Autodesk Inventor part; units mm, degrees
(part 3 of 3)
sketch "Sketch7" plane through (0, 0, 2.286) normal (0, 0, 1) x (1, 0, 0)
  arc A0 (-117.475, -252.4125) -> (-119.38, -258.1275) centre (-117.475, -255.5875) ccw projected
  line L0 (-79.375, -252.4125) -> (-117.475, -252.4125) projected
  arc A1 (-76.2, -255.5875) -> (-79.375, -252.4125) centre (-79.375, -255.5875) ccw projected
  line L1 (-76.2, -284.1625) -> (-76.2, -255.5875) projected
  arc A2 (-81.28, -286.7025) -> (-76.2, -284.1625) centre (-79.375, -284.1625) ccw projected
  line L2 (-119.38, -258.1275) -> (-81.28, -286.7025) projected
  arc A3 (-127, 290.5125) -> (-121.92, 287.9725) centre (-123.825, 290.5125) ccw projected
  line L3 (-127, 319.0875) -> (-127, 290.5125) projected
  arc A4 (-123.825, 322.2625) -> (-127, 319.0875) centre (-123.825, 319.0875) ccw projected
  line L4 (-85.725, 322.2625) -> (-123.825, 322.2625) projected
  arc A5 (-83.82, 316.5475) -> (-85.725, 322.2625) centre (-85.725, 319.0875) ccw projected
  line L5 (-121.92, 287.9725) -> (-83.82, 316.5475) projected
  arc A6 (-180.975, 322.2625) -> (-182.88, 316.5475) centre (-180.975, 319.0875) ccw projected
  line L6 (-142.875, 322.2625) -> (-180.975, 322.2625) projected
  arc A7 (-139.7, 319.0875) -> (-142.875, 322.2625) centre (-142.875, 319.0875) ccw projected
  line L7 (-139.7, 290.5125) -> (-139.7, 319.0875) projected
  arc A8 (-144.78, 287.9725) -> (-139.7, 290.5125) centre (-142.875, 290.5125) ccw projected
  line L8 (-182.88, 316.5475) -> (-144.78, 287.9725) projected
  arc A9 (-142.875, 201.6125) -> (-139.7, 204.7875) centre (-142.875, 204.7875) ccw projected
  line L9 (-180.975, 201.6125) -> (-142.875, 201.6125) projected
  arc A10 (-182.88, 207.3275) -> (-180.975, 201.6125) centre (-180.975, 204.7875) ccw projected
  line L10 (-144.78, 235.9025) -> (-182.88, 207.3275) projected
  arc A11 (-139.7, 233.3625) -> (-144.78, 235.9025) centre (-142.875, 233.3625) ccw projected
  line L11 (-139.7, 204.7875) -> (-139.7, 233.3625) projected
  arc A12 (-85.725, 201.6125) -> (-83.82, 207.3275) centre (-85.725, 204.7875) ccw projected
  line L12 (-123.825, 201.6125) -> (-85.725, 201.6125) projected
  arc A13 (-127, 204.7875) -> (-123.825, 201.6125) centre (-123.825, 204.7875) ccw projected
  line L13 (-127, 233.3625) -> (-127, 204.7875) projected
  arc A14 (-121.92, 235.9025) -> (-127, 233.3625) centre (-123.825, 233.3625) ccw projected
  line L14 (-83.82, 207.3275) -> (-121.92, 235.9025) projected
  arc A15 (200.025, 322.2625) -> (198.12, 316.5475) centre (200.025, 319.0875) ccw projected
  line L15 (238.125, 322.2625) -> (200.025, 322.2625) projected
  arc A16 (241.3, 319.0875) -> (238.125, 322.2625) centre (238.125, 319.0875) ccw projected
  line L16 (241.3, 290.5125) -> (241.3, 319.0875) projected
  arc A17 (236.22, 287.9725) -> (241.3, 290.5125) centre (238.125, 290.5125) ccw projected
  line L17 (198.12, 316.5475) -> (236.22, 287.9725) projected
  arc A18 (-190.5, 271.4625) -> (-187.325, 268.2875) centre (-187.325, 271.4625) ccw projected
  line L18 (-190.5, 300.0375) -> (-190.5, 271.4625) projected
  arc A19 (-185.42, 302.5775) -> (-190.5, 300.0375) centre (-187.325, 300.0375) ccw projected
  line L19 (-147.32, 274.0025) -> (-185.42, 302.5775) projected
  arc A20 (-149.225, 268.2875) -> (-147.32, 274.0025) centre (-149.225, 271.4625) ccw projected
  line L20 (-187.325, 268.2875) -> (-149.225, 268.2875) projected
  arc A21 (-76.2, 300.0375) -> (-81.28, 302.5775) centre (-79.375, 300.0375) ccw projected
  line L21 (-76.2, 271.4625) -> (-76.2, 300.0375) projected
  arc A22 (-79.375, 268.2875) -> (-76.2, 271.4625) centre (-79.375, 271.4625) ccw projected
  line L22 (-117.475, 268.2875) -> (-79.375, 268.2875) projected
  arc A23 (-119.38, 274.0025) -> (-117.475, 268.2875) centre (-117.475, 271.4625) ccw projected
  line L23 (-81.28, 302.5775) -> (-119.38, 274.0025) projected
  arc A24 (238.125, 201.6125) -> (241.3, 204.7875) centre (238.125, 204.7875) ccw projected
  line L24 (200.025, 201.6125) -> (238.125, 201.6125) projected
  arc A25 (198.12, 207.3275) -> (200.025, 201.6125) centre (200.025, 204.7875) ccw projected
  line L25 (236.22, 235.9025) -> (198.12, 207.3275) projected
  arc A26 (241.3, 233.3625) -> (236.22, 235.9025) centre (238.125, 233.3625) ccw projected
  line L26 (241.3, 204.7875) -> (241.3, 233.3625) projected
  arc A27 (233.68, 249.8725) -> (231.775, 255.5875) centre (231.775, 252.4125) ccw projected
  line L27 (195.58, 221.2975) -> (233.68, 249.8725) projected
  arc A28 (190.5, 223.8375) -> (195.58, 221.2975) centre (193.675, 223.8375) ccw projected
  line L28 (190.5, 252.4125) -> (190.5, 223.8375) projected
  arc A29 (193.675, 255.5875) -> (190.5, 252.4125) centre (193.675, 252.4125) ccw projected
  line L29 (231.775, 255.5875) -> (193.675, 255.5875) projected
  arc A30 (-149.225, -373.0625) -> (-147.32, -367.3475) centre (-149.225, -369.8875) ccw projected
  line L30 (-187.325, -373.0625) -> (-149.225, -373.0625) projected
  arc A31 (-190.5, -369.8875) -> (-187.325, -373.0625) centre (-187.325, -369.8875) ccw projected
  line L31 (-190.5, -341.3125) -> (-190.5, -369.8875) projected
  arc A32 (-185.42, -338.7725) -> (-190.5, -341.3125) centre (-187.325, -341.3125) ccw projected
  line L32 (-147.32, -367.3475) -> (-185.42, -338.7725) projected
  arc A33 (-119.38, -367.3475) -> (-117.475, -373.0625) centre (-117.475, -369.8875) ccw projected
  line L33 (-81.28, -338.7725) -> (-119.38, -367.3475) projected
  arc A34 (-76.2, -341.3125) -> (-81.28, -338.7725) centre (-79.375, -341.3125) ccw projected
  line L34 (-76.2, -369.8875) -> (-76.2, -341.3125) projected
  arc A35 (-79.375, -373.0625) -> (-76.2, -369.8875) centre (-79.375, -369.8875) ccw projected
  line L35 (-117.475, -373.0625) -> (-79.375, -373.0625) projected
  arc A36 (127, 290.5125) -> (132.08, 287.9725) centre (130.175, 290.5125) ccw projected
  line L36 (127, 319.0875) -> (127, 290.5125) projected
  arc A37 (130.175, 322.2625) -> (127, 319.0875) centre (130.175, 319.0875) ccw projected
  line L37 (168.275, 322.2625) -> (130.175, 322.2625) projected
  arc A38 (170.18, 316.5475) -> (168.275, 322.2625) centre (168.275, 319.0875) ccw projected
  line L38 (132.08, 287.9725) -> (170.18, 316.5475) projected
  arc A39 (132.08, 235.9025) -> (127, 233.3625) centre (130.175, 233.3625) ccw projected
  line L39 (170.18, 207.3275) -> (132.08, 235.9025) projected
  arc A40 (168.275, 201.6125) -> (170.18, 207.3275) centre (168.275, 204.7875) ccw projected
  line L40 (130.175, 201.6125) -> (168.275, 201.6125) projected
  arc A41 (127, 204.7875) -> (130.175, 201.6125) centre (130.175, 204.7875) ccw projected
  line L41 (127, 233.3625) -> (127, 204.7875) projected
  arc A42 (177.8, 300.0375) -> (172.72, 302.5775) centre (174.625, 300.0375) ccw projected
  line L42 (177.8, 271.4625) -> (177.8, 300.0375) projected
  arc A43 (174.625, 268.2875) -> (177.8, 271.4625) centre (174.625, 271.4625) ccw projected
  line L43 (136.525, 268.2875) -> (174.625, 268.2875) projected
  arc A44 (134.62, 274.0025) -> (136.525, 268.2875) centre (136.525, 271.4625) ccw projected
  line L44 (172.72, 302.5775) -> (134.62, 274.0025) projected
  arc A45 (195.58, 302.5775) -> (190.5, 300.0375) centre (193.675, 300.0375) ccw projected
  line L45 (233.68, 274.0025) -> (195.58, 302.5775) projected
  arc A46 (231.775, 268.2875) -> (233.68, 274.0025) centre (231.775, 271.4625) ccw projected
  line L46 (193.675, 268.2875) -> (231.775, 268.2875) projected
  arc A47 (190.5, 271.4625) -> (193.675, 268.2875) centre (193.675, 271.4625) ccw projected
  line L47 (190.5, 300.0375) -> (190.5, 271.4625) projected
  arc A48 (172.72, 221.2975) -> (177.8, 223.8375) centre (174.625, 223.8375) ccw projected
  line L48 (134.62, 249.8725) -> (172.72, 221.2975) projected
  arc A49 (136.525, 255.5875) -> (134.62, 249.8725) centre (136.525, 252.4125) ccw projected
  line L49 (174.625, 255.5875) -> (136.525, 255.5875) projected
  arc A50 (177.8, 252.4125) -> (174.625, 255.5875) centre (174.625, 252.4125) ccw projected
  line L50 (177.8, 223.8375) -> (177.8, 252.4125) projected
  arc A51 (-190.5, 223.8375) -> (-185.42, 221.2975) centre (-187.325, 223.8375) ccw projected
  line L51 (-190.5, 252.4125) -> (-190.5, 223.8375) projected
  arc A52 (-187.325, 255.5875) -> (-190.5, 252.4125) centre (-187.325, 252.4125) ccw projected
  line L52 (-149.225, 255.5875) -> (-187.325, 255.5875) projected
  arc A53 (-147.32, 249.8725) -> (-149.225, 255.5875) centre (-149.225, 252.4125) ccw projected
  line L53 (-185.42, 221.2975) -> (-147.32, 249.8725) projected
  arc A54 (-144.78, -353.3775) -> (-139.7, -350.8375) centre (-142.875, -350.8375) ccw projected
  line L54 (-182.88, -324.8025) -> (-144.78, -353.3775) projected
  arc A55 (-180.975, -319.0875) -> (-182.88, -324.8025) centre (-180.975, -322.2625) ccw projected
  line L55 (-142.875, -319.0875) -> (-180.975, -319.0875) projected
  arc A56 (-139.7, -322.2625) -> (-142.875, -319.0875) centre (-142.875, -322.2625) ccw projected
  line L56 (-139.7, -350.8375) -> (-139.7, -322.2625) projected
  arc A57 (-123.825, -319.0875) -> (-127, -322.2625) centre (-123.825, -322.2625) ccw projected
  line L57 (-85.725, -319.0875) -> (-123.825, -319.0875) projected
  arc A58 (-83.82, -324.8025) -> (-85.725, -319.0875) centre (-85.725, -322.2625) ccw projected
  line L58 (-121.92, -353.3775) -> (-83.82, -324.8025) projected
  arc A59 (-127, -350.8375) -> (-121.92, -353.3775) centre (-123.825, -350.8375) ccw projected
  line L59 (-127, -322.2625) -> (-127, -350.8375) projected
  arc A60 (-81.28, 221.2975) -> (-76.2, 223.8375) centre (-79.375, 223.8375) ccw projected
  line L60 (-119.38, 249.8725) -> (-81.28, 221.2975) projected
  arc A61 (-117.475, 255.5875) -> (-119.38, 249.8725) centre (-117.475, 252.4125) ccw projected
  line L61 (-79.375, 255.5875) -> (-117.475, 255.5875) projected
  arc A62 (-76.2, 252.4125) -> (-79.375, 255.5875) centre (-79.375, 252.4125) ccw projected
  line L62 (-76.2, 223.8375) -> (-76.2, 252.4125) projected
  arc A63 (-142.875, -306.3875) -> (-139.7, -303.2125) centre (-142.875, -303.2125) ccw projected
  line L63 (-180.975, -306.3875) -> (-142.875, -306.3875) projected
  arc A64 (-182.88, -300.6725) -> (-180.975, -306.3875) centre (-180.975, -303.2125) ccw projected
  line L64 (-144.78, -272.0975) -> (-182.88, -300.6725) projected
  arc A65 (-139.7, -274.6375) -> (-144.78, -272.0975) centre (-142.875, -274.6375) ccw projected
  line L65 (-139.7, -303.2125) -> (-139.7, -274.6375) projected
  arc A66 (-190.5, -284.1625) -> (-185.42, -286.7025) centre (-187.325, -284.1625) ccw projected
  line L66 (-190.5, -255.5875) -> (-190.5, -284.1625) projected
  arc A67 (-187.325, -252.4125) -> (-190.5, -255.5875) centre (-187.325, -255.5875) ccw projected
  line L67 (-149.225, -252.4125) -> (-187.325, -252.4125) projected
  arc A68 (-147.32, -258.1275) -> (-149.225, -252.4125) centre (-149.225, -255.5875) ccw projected
  line L68 (-185.42, -286.7025) -> (-147.32, -258.1275) projected
  arc A69 (177.8, -341.3125) -> (172.72, -338.7725) centre (174.625, -341.3125) ccw projected
  line L69 (177.8, -369.8875) -> (177.8, -341.3125) projected
  arc A70 (174.625, -373.0625) -> (177.8, -369.8875) centre (174.625, -369.8875) ccw projected
  line L70 (136.525, -373.0625) -> (174.625, -373.0625) projected
  arc A71 (134.62, -367.3475) -> (136.525, -373.0625) centre (136.525, -369.8875) ccw projected
  line L71 (172.72, -338.7725) -> (134.62, -367.3475) projected
  arc A72 (-85.725, -306.3875) -> (-83.82, -300.6725) centre (-85.725, -303.2125) ccw projected
  line L72 (-123.825, -306.3875) -> (-85.725, -306.3875) projected
  arc A73 (-127, -303.2125) -> (-123.825, -306.3875) centre (-123.825, -303.2125) ccw projected
  line L73 (-127, -274.6375) -> (-127, -303.2125) projected
  arc A74 (-121.92, -272.0975) -> (-127, -274.6375) centre (-123.825, -274.6375) ccw projected
  line L74 (-83.82, -300.6725) -> (-121.92, -272.0975) projected
  arc A75 (136.525, -252.4125) -> (134.62, -258.1275) centre (136.525, -255.5875) ccw projected
  line L75 (174.625, -252.4125) -> (136.525, -252.4125) projected
  arc A76 (177.8, -255.5875) -> (174.625, -252.4125) centre (174.625, -255.5875) ccw projected
  line L76 (177.8, -284.1625) -> (177.8, -255.5875) projected
  arc A77 (172.72, -286.7025) -> (177.8, -284.1625) centre (174.625, -284.1625) ccw projected
  line L77 (134.62, -258.1275) -> (172.72, -286.7025) projected
  arc A78 (132.08, -272.0975) -> (127, -274.6375) centre (130.175, -274.6375) ccw projected
  line L78 (170.18, -300.6725) -> (132.08, -272.0975) projected
  arc A79 (168.275, -306.3875) -> (170.18, -300.6725) centre (168.275, -303.2125) ccw projected
  line L79 (130.175, -306.3875) -> (168.275, -306.3875) projected
  arc A80 (127, -303.2125) -> (130.175, -306.3875) centre (130.175, -303.2125) ccw projected
  line L80 (127, -274.6375) -> (127, -303.2125) projected
  arc A81 (233.68, -258.1275) -> (231.775, -252.4125) centre (231.775, -255.5875) ccw projected
  line L81 (195.58, -286.7025) -> (233.68, -258.1275) projected
  arc A82 (190.5, -284.1625) -> (195.58, -286.7025) centre (193.675, -284.1625) ccw projected
  line L82 (190.5, -255.5875) -> (190.5, -284.1625) projected
  arc A83 (193.675, -252.4125) -> (190.5, -255.5875) centre (193.675, -255.5875) ccw projected
  line L83 (231.775, -252.4125) -> (193.675, -252.4125) projected
  arc A84 (198.12, -300.6725) -> (200.025, -306.3875) centre (200.025, -303.2125) ccw projected
  line L84 (236.22, -272.0975) -> (198.12, -300.6725) projected
  arc A85 (241.3, -274.6375) -> (236.22, -272.0975) centre (238.125, -274.6375) ccw projected
  line L85 (241.3, -303.2125) -> (241.3, -274.6375) projected
  arc A86 (238.125, -306.3875) -> (241.3, -303.2125) centre (238.125, -303.2125) ccw projected
  line L86 (200.025, -306.3875) -> (238.125, -306.3875) projected
  arc A87 (127, -350.8375) -> (132.08, -353.3775) centre (130.175, -350.8375) ccw projected
  line L87 (127, -322.2625) -> (127, -350.8375) projected
  arc A88 (130.175, -319.0875) -> (127, -322.2625) centre (130.175, -322.2625) ccw projected
  line L88 (168.275, -319.0875) -> (130.175, -319.0875) projected
  arc A89 (170.18, -324.8025) -> (168.275, -319.0875) centre (168.275, -322.2625) ccw projected
  line L89 (132.08, -353.3775) -> (170.18, -324.8025) projected
  arc A90 (195.58, -338.7725) -> (190.5, -341.3125) centre (193.675, -341.3125) ccw projected
  line L90 (233.68, -367.3475) -> (195.58, -338.7725) projected
  arc A91 (231.775, -373.0625) -> (233.68, -367.3475) centre (231.775, -369.8875) ccw projected
  line L91 (193.675, -373.0625) -> (231.775, -373.0625) projected
  arc A92 (190.5, -369.8875) -> (193.675, -373.0625) centre (193.675, -369.8875) ccw projected
  line L92 (190.5, -341.3125) -> (190.5, -369.8875) projected
  arc A93 (200.025, -319.0875) -> (198.12, -324.8025) centre (200.025, -322.2625) ccw projected
  line L93 (238.125, -319.0875) -> (200.025, -319.0875) projected
  arc A94 (241.3, -322.2625) -> (238.125, -319.0875) centre (238.125, -322.2625) ccw projected
  line L94 (241.3, -350.8375) -> (241.3, -322.2625) projected
  arc A95 (236.22, -353.3775) -> (241.3, -350.8375) centre (238.125, -350.8375) ccw projected
  line L95 (198.12, -324.8025) -> (236.22, -353.3775) projected
  line L96 (-187.325, 322.2625) -> (-79.375, 322.2625)
  line L97 (-76.2, 319.0875) -> (-76.2, 204.7875)
  line L98 (-79.375, 201.6125) -> (-187.325, 201.6125)
  line L99 (-190.5, 204.7875) -> (-190.5, 319.0875)
  line L100 (130.175, 322.2625) -> (238.125, 322.2625)
  line L101 (241.3, 319.0875) -> (241.3, 204.7875)
  line L102 (238.125, 201.6125) -> (130.175, 201.6125)
  line L103 (127, 204.7875) -> (127, 319.0875)
  arc A96 (-187.325, 322.2625) -> (-190.5, 319.0875) centre (-187.325, 319.0875) ccw
  arc A97 (-190.5, 204.7875) -> (-187.325, 201.6125) centre (-187.325, 204.7875) ccw
  arc A98 (-79.375, 201.6125) -> (-76.2, 204.7875) centre (-79.375, 204.7875) ccw
  arc A99 (-76.2, 319.0875) -> (-79.375, 322.2625) centre (-79.375, 319.0875) ccw
  arc A100 (130.175, 322.2625) -> (127, 319.0875) centre (130.175, 319.0875) ccw
  arc A101 (241.3, 319.0875) -> (238.125, 322.2625) centre (238.125, 319.0875) ccw
  arc A102 (238.125, 201.6125) -> (241.3, 204.7875) centre (238.125, 204.7875) ccw
  arc A103 (127, 204.7875) -> (130.175, 201.6125) centre (130.175, 204.7875) ccw
  line L104 (-187.325, -252.4125) -> (-79.375, -252.4125)
  line L105 (-76.2, -255.5875) -> (-76.2, -369.8875)
  line L106 (-79.375, -373.0625) -> (-187.325, -373.0625)
  line L107 (-190.5, -369.8875) -> (-190.5, -255.5875)
  line L108 (130.175, -252.4125) -> (238.125, -252.4125)
  line L109 (241.3, -255.5875) -> (241.3, -369.8875)
  line L110 (238.125, -373.0625) -> (130.175, -373.0625)
  line L111 (127, -369.8875) -> (127, -255.5875)
  arc A104 (-187.325, -252.4125) -> (-190.5, -255.5875) centre (-187.325, -255.5875) ccw
  arc A105 (-190.5, -369.8875) -> (-187.325, -373.0625) centre (-187.325, -369.8875) ccw
  arc A106 (-79.375, -373.0625) -> (-76.2, -369.8875) centre (-79.375, -369.8875) ccw
  arc A107 (-76.2, -255.5875) -> (-79.375, -252.4125) centre (-79.375, -255.5875) ccw
  arc A108 (130.175, -252.4125) -> (127, -255.5875) centre (130.175, -255.5875) ccw
  arc A109 (127, -369.8875) -> (130.175, -373.0625) centre (130.175, -369.8875) ccw
  arc A110 (238.125, -373.0625) -> (241.3, -369.8875) centre (238.125, -369.8875) ccw
  arc A111 (241.3, -255.5875) -> (238.125, -252.4125) centre (238.125, -255.5875) ccw
  point P0 (0, 0)
  dimension "d349" = 0
  dimension "d350" = 0
  dimension "d351" = 0
  dimension "d352" = 0
  dimension "d353" = 0
  dimension "d354" = 0
  dimension "d355" = 0
  dimension "d356" = 0
  dimension "d357" = 3.175
  dimension "d358" = 0
  dimension "d359" = 0
  dimension "d360" = 0
  dimension "d361" = 0
  dimension "d362" = 0
  dimension "d363" = 0
  dimension "d364" = 0
  dimension "d365" = 0
  dimension "d366" = 3.175
  constraints: 32 end point, 32 point on circle, 32 tangent, 16 centre point, 14 equal radius, 8 parallel, 4 horizontal, 4 perpendicular
  measures "d349" distance between parallel lines of L18 L99
  measures "d350" distance between parallel lines of L6 L96
  measures "d351" distance between parallel lines of L21 L97
  measures "d352" distance between parallel lines of L9 L98
  measures "d353" distance between parallel lines of L26 L101
  measures "d354" distance between parallel lines of L40 L102
  measures "d355" distance between parallel lines of L41 L103
  measures "d356" distance between parallel lines of L37 L100
  measures "d357" radius of A96
  measures "d358" distance between parallel lines of L1 L105
  measures "d359" distance between parallel lines of L30 L106
  measures "d360" distance between parallel lines of L66 L107
  measures "d361" distance between parallel lines of L67 L104
  measures "d362" distance between parallel lines of L85 L109
  measures "d363" distance between parallel lines of L75 L108
  measures "d364" distance between parallel lines of L80 L111
  measures "d365" distance between parallel lines of L70 L110
  measures "d366" radius of A104
extrude "Extrusion5" cut sketch "Sketch7" against normal blind 25.4 contours A0 L2 A2 L105 A34 L33 A33 L106 A30 L32 A32 L107 A66 L68 A68 L104 | A3 L5 A5 L96 A99 L97 A21 L23 A23 L22 A22 A62 L61 A61 L60 A60 A98 L98 A12 L14 A14 L13 A13 A9 L11 A11 L10 A10 A97 L99 A51 L53 A53 L52 A52 A18 L20 A20 L19 A19 A96 A6 L8 A8 L7 A7 A4 L3 | A15 L17 A17 L101 A26 L25 A25 L102 A40 L39 A39 L103 A36 L38 A38 L100 | A69 L71 A71 L110 A109 L111 A87 L89 A89 L88 A88 A80 L79 A79 L78 A78 A108 L108 A75 L77 A77 L76 A76 A83 L82 A82 L81 A81 A111 L109 A85 L84 A84 L86 A86 A94 L93 A93 L95 A95 A110 A91 L90 A90 L92 A92 A70 L69
sketch "Sketch8" plane through (0, 0, 2.286) normal (0, 0, 1) x (1, 0, 0)
  arc A0 (195.58, -205.4225) -> (190.5, -207.9625) centre (193.675, -207.9625) ccw projected
  line L0 (233.68, -233.9975) -> (195.58, -205.4225) projected
  arc A1 (231.775, -239.7125) -> (233.68, -233.9975) centre (231.775, -236.5375) ccw projected
  line L1 (193.675, -239.7125) -> (231.775, -239.7125) projected
  arc A2 (190.5, -236.5375) -> (193.675, -239.7125) centre (193.675, -236.5375) ccw projected
  line L2 (190.5, -207.9625) -> (190.5, -236.5375) projected
  arc A3 (200.025, -185.7375) -> (198.12, -191.4525) centre (200.025, -188.9125) ccw projected
  line L3 (238.125, -185.7375) -> (200.025, -185.7375) projected
  arc A4 (241.3, -188.9125) -> (238.125, -185.7375) centre (238.125, -188.9125) ccw projected
  line L4 (241.3, -217.4875) -> (241.3, -188.9125) projected
  arc A5 (236.22, -220.0275) -> (241.3, -217.4875) centre (238.125, -217.4875) ccw projected
  line L5 (198.12, -191.4525) -> (236.22, -220.0275) projected
  arc A6 (170.18, -191.4525) -> (168.275, -185.7375) centre (168.275, -188.9125) ccw projected
  line L6 (132.08, -220.0275) -> (170.18, -191.4525) projected
  arc A7 (127, -217.4875) -> (132.08, -220.0275) centre (130.175, -217.4875) ccw projected
  line L7 (127, -188.9125) -> (127, -217.4875) projected
  arc A8 (130.175, -185.7375) -> (127, -188.9125) centre (130.175, -188.9125) ccw projected
  line L8 (168.275, -185.7375) -> (130.175, -185.7375) projected
  arc A9 (134.62, -233.9975) -> (136.525, -239.7125) centre (136.525, -236.5375) ccw projected
  line L9 (172.72, -205.4225) -> (134.62, -233.9975) projected
  arc A10 (177.8, -207.9625) -> (172.72, -205.4225) centre (174.625, -207.9625) ccw projected
  line L10 (177.8, -236.5375) -> (177.8, -207.9625) projected
  arc A11 (174.625, -239.7125) -> (177.8, -236.5375) centre (174.625, -236.5375) ccw projected
  line L11 (136.525, -239.7125) -> (174.625, -239.7125) projected
  arc A12 (-185.42, -205.4225) -> (-190.5, -207.9625) centre (-187.325, -207.9625) ccw projected
  line L12 (-147.32, -233.9975) -> (-185.42, -205.4225) projected
  arc A13 (-149.225, -239.7125) -> (-147.32, -233.9975) centre (-149.225, -236.5375) ccw projected
  line L13 (-187.325, -239.7125) -> (-149.225, -239.7125) projected
  arc A14 (-190.5, -236.5375) -> (-187.325, -239.7125) centre (-187.325, -236.5375) ccw projected
  line L14 (-190.5, -207.9625) -> (-190.5, -236.5375) projected
  arc A15 (-139.7, -188.9125) -> (-142.875, -185.7375) centre (-142.875, -188.9125) ccw projected
  line L15 (-139.7, -217.4875) -> (-139.7, -188.9125) projected
  arc A16 (-144.78, -220.0275) -> (-139.7, -217.4875) centre (-142.875, -217.4875) ccw projected
  line L16 (-182.88, -191.4525) -> (-144.78, -220.0275) projected
  arc A17 (-180.975, -185.7375) -> (-182.88, -191.4525) centre (-180.975, -188.9125) ccw projected
  line L17 (-142.875, -185.7375) -> (-180.975, -185.7375) projected
  arc A18 (-119.38, -233.9975) -> (-117.475, -239.7125) centre (-117.475, -236.5375) ccw projected
  line L18 (-81.28, -205.4225) -> (-119.38, -233.9975) projected
  arc A19 (-76.2, -207.9625) -> (-81.28, -205.4225) centre (-79.375, -207.9625) ccw projected
  line L19 (-76.2, -236.5375) -> (-76.2, -207.9625) projected
  arc A20 (-79.375, -239.7125) -> (-76.2, -236.5375) centre (-79.375, -236.5375) ccw projected
  line L20 (-117.475, -239.7125) -> (-79.375, -239.7125) projected
  arc A21 (-127, -217.4875) -> (-121.92, -220.0275) centre (-123.825, -217.4875) ccw projected
  line L21 (-127, -188.9125) -> (-127, -217.4875) projected
  arc A22 (-123.825, -185.7375) -> (-127, -188.9125) centre (-123.825, -188.9125) ccw projected
  line L22 (-85.725, -185.7375) -> (-123.825, -185.7375) projected
  arc A23 (-83.82, -191.4525) -> (-85.725, -185.7375) centre (-85.725, -188.9125) ccw projected
  line L23 (-121.92, -220.0275) -> (-83.82, -191.4525) projected
  arc A24 (-149.225, 134.9375) -> (-147.32, 140.6525) centre (-149.225, 138.1125) ccw projected
  line L24 (-187.325, 134.9375) -> (-149.225, 134.9375) projected
  arc A25 (-190.5, 138.1125) -> (-187.325, 134.9375) centre (-187.325, 138.1125) ccw projected
  line L25 (-190.5, 166.6875) -> (-190.5, 138.1125) projected
  arc A26 (-185.42, 169.2275) -> (-190.5, 166.6875) centre (-187.325, 166.6875) ccw projected
  line L26 (-147.32, 140.6525) -> (-185.42, 169.2275) projected
  arc A27 (134.62, 140.6525) -> (136.525, 134.9375) centre (136.525, 138.1125) ccw projected
  line L27 (172.72, 169.2275) -> (134.62, 140.6525) projected
  arc A28 (177.8, 166.6875) -> (172.72, 169.2275) centre (174.625, 166.6875) ccw projected
  line L28 (177.8, 138.1125) -> (177.8, 166.6875) projected
  arc A29 (174.625, 134.9375) -> (177.8, 138.1125) centre (174.625, 138.1125) ccw projected
  line L29 (136.525, 134.9375) -> (174.625, 134.9375) projected
  arc A30 (-79.375, 134.9375) -> (-76.2, 138.1125) centre (-79.375, 138.1125) ccw projected
  line L30 (-117.475, 134.9375) -> (-79.375, 134.9375) projected
  arc A31 (-119.38, 140.6525) -> (-117.475, 134.9375) centre (-117.475, 138.1125) ccw projected
  line L31 (-81.28, 169.2275) -> (-119.38, 140.6525) projected
  arc A32 (-76.2, 166.6875) -> (-81.28, 169.2275) centre (-79.375, 166.6875) ccw projected
  line L32 (-76.2, 138.1125) -> (-76.2, 166.6875) projected
  arc A33 (130.175, 188.9125) -> (127, 185.7375) centre (130.175, 185.7375) ccw projected
  line L33 (168.275, 188.9125) -> (130.175, 188.9125) projected
  arc A34 (170.18, 183.1975) -> (168.275, 188.9125) centre (168.275, 185.7375) ccw projected
  line L34 (132.08, 154.6225) -> (170.18, 183.1975) projected
  arc A35 (127, 157.1625) -> (132.08, 154.6225) centre (130.175, 157.1625) ccw projected
  line L35 (127, 185.7375) -> (127, 157.1625) projected
  arc A36 (200.025, 188.9125) -> (198.12, 183.1975) centre (200.025, 185.7375) ccw projected
  line L36 (238.125, 188.9125) -> (200.025, 188.9125) projected
  arc A37 (241.3, 185.7375) -> (238.125, 188.9125) centre (238.125, 185.7375) ccw projected
  line L37 (241.3, 157.1625) -> (241.3, 185.7375) projected
  arc A38 (236.22, 154.6225) -> (241.3, 157.1625) centre (238.125, 157.1625) ccw projected
  line L38 (198.12, 183.1975) -> (236.22, 154.6225) projected
  arc A39 (231.775, 134.9375) -> (233.68, 140.6525) centre (231.775, 138.1125) ccw projected
  line L39 (193.675, 134.9375) -> (231.775, 134.9375) projected
  arc A40 (190.5, 138.1125) -> (193.675, 134.9375) centre (193.675, 138.1125) ccw projected
  line L40 (190.5, 166.6875) -> (190.5, 138.1125) projected
  arc A41 (195.58, 169.2275) -> (190.5, 166.6875) centre (193.675, 166.6875) ccw projected
  line L41 (233.68, 140.6525) -> (195.58, 169.2275) projected
  arc A42 (-127, 157.1625) -> (-121.92, 154.6225) centre (-123.825, 157.1625) ccw projected
  line L42 (-127, 185.7375) -> (-127, 157.1625) projected
  arc A43 (-123.825, 188.9125) -> (-127, 185.7375) centre (-123.825, 185.7375) ccw projected
  line L43 (-85.725, 188.9125) -> (-123.825, 188.9125) projected
  arc A44 (-83.82, 183.1975) -> (-85.725, 188.9125) centre (-85.725, 185.7375) ccw projected
  line L44 (-121.92, 154.6225) -> (-83.82, 183.1975) projected
  arc A45 (-139.7, 185.7375) -> (-142.875, 188.9125) centre (-142.875, 185.7375) ccw projected
  line L45 (-139.7, 157.1625) -> (-139.7, 185.7375) projected
  arc A46 (-144.78, 154.6225) -> (-139.7, 157.1625) centre (-142.875, 157.1625) ccw projected
  line L46 (-182.88, 183.1975) -> (-144.78, 154.6225) projected
  arc A47 (-180.975, 188.9125) -> (-182.88, 183.1975) centre (-180.975, 185.7375) ccw projected
  line L47 (-142.875, 188.9125) -> (-180.975, 188.9125) projected
  point P0 (0, 0)
extrude "Extrusion6" add sketch "Sketch8" against normal blind 2.286
sketch "Sketch9" plane through (0, 0, 2.286) normal (0, 0, 1) x (1, 0, 0)
  line L0 (-171.45, -101.6) -> (-228.6, -101.6) projected
  line L1 (279.4, -457.2) -> (-228.6, -457.2) projected
  line L2 (222.25, -101.6) -> (222.25, 50.8) projected
  line L3 (-228.6, 406.4) -> (279.4, 406.4) projected
  line L4 (-171.45, 50.8) -> (-171.45, -101.6) projected
  line L5 (-190.5, 204.7875) -> (-190.5, 319.0875) projected
  line L6 (-79.375, 201.6125) -> (-187.325, 201.6125) projected
  line L7 (-158.75, 171.45) -> (-107.95, 171.45) construction
  line L8 (-158.75, 184.15) -> (-107.95, 184.15)
  line L9 (-107.95, 158.75) -> (-158.75, 158.75)
  arc A0 (-158.75, 184.15) -> (-158.75, 158.75) centre (-158.75, 171.45) ccw
  arc A1 (-107.95, 158.75) -> (-107.95, 184.15) centre (-107.95, 171.45) ccw
  line L10 (-171.45, -25.4) -> (222.25, -25.4) construction
  line L11 (25.4, 406.4) -> (25.4, -457.2) construction
  line L12 (209.55, 171.45) -> (158.75, 171.45) construction
  line L13 (209.55, 184.15) -> (158.75, 184.15)
  line L14 (158.75, 158.75) -> (209.55, 158.75)
  arc A2 (209.55, 158.75) -> (209.55, 184.15) centre (209.55, 171.45) ccw
  arc A3 (158.75, 184.15) -> (158.75, 158.75) centre (158.75, 171.45) ccw
  line L15 (-158.75, -222.25) -> (-107.95, -222.25) construction
  line L16 (-158.75, -234.95) -> (-107.95, -234.95)
  line L17 (-107.95, -209.55) -> (-158.75, -209.55)
  arc A4 (-158.75, -209.55) -> (-158.75, -234.95) centre (-158.75, -222.25) ccw
  arc A5 (-107.95, -234.95) -> (-107.95, -209.55) centre (-107.95, -222.25) ccw
  line L18 (209.55, -234.95) -> (158.75, -234.95)
  line L19 (209.55, -222.25) -> (158.75, -222.25) construction
  line L20 (158.75, -209.55) -> (209.55, -209.55)
  arc A6 (158.75, -209.55) -> (158.75, -234.95) centre (158.75, -222.25) ccw
  arc A7 (209.55, -234.95) -> (209.55, -209.55) centre (209.55, -222.25) ccw
  point P0 (0, 0)
  point P1 (-133.35, 171.45)
  point P2 (184.15, 171.45)
  point P3 (-133.35, -222.25)
  point P4 (184.15, -222.25)
  dimension "d371" = 50.8
  dimension "d372" = 57.15
  dimension "d373" = 25.4
  dimension "d374" = 30.1625
  constraints: 36 end point, 21 symmetric about line, 16 point on circle, 8 centre point, 5 midpoint, 4 tangent, 2 parallel, 6 other
  measures "d371" distance of L7.start L7.end
  measures "d372" distance from line of L5 point (-133.35, 171.45)
  measures "d373" distance between parallel lines of L9 L8
  measures "d374" distance from line of L6 point (-133.35, 171.45)
extrude "Extrusion7" cut sketch "Sketch9" against normal blind 2.286
fillet "Fillet1" radius 3.175 28 edges at (-171.45, 50.8, 1.143) (-228.6, 76.2, 1.143) (-171.45, -101.6, 1.143) (-228.6, -127, 1.143) (-228.6, -203.2, 1.143) (-228.6, 152.4, 1.143) (222.25, 50.8, 1.143) (222.25, -101.6, 1.143) (279.4, 76.2, 1.143) (279.4, 152.4, 1.143) (279.4, -127, 1.143) (279.4, -203.2, 1.143) (-330.2, 152.4, 1.143) (-330.2, 76.2, 1.143) (-228.6, 50.8, 1.143) (-228.6, -101.6, 1.143) (-330.2, -127, 1.143) (-330.2, -203.2, 1.143) (-228.6, -457.2, 1.143) (279.4, -457.2, 1.143) (381, -203.2, 1.143) (381, -127, 1.143) (279.4, -101.6, 1.143) (279.4, 50.8, 1.143) (381, 76.2, 1.143) (381, 152.4, 1.143) (279.4, 406.4, 1.143) (-228.6, 406.4, 1.143)
equation "\"d9\" = d8"
equation "\"d10\" = d7"
equation "\"d18\" = d7"
equation "\"d19\" = d18"
body "Solid1"
